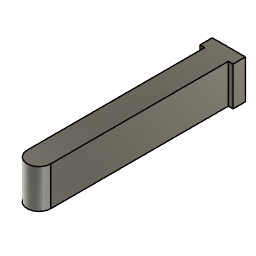
ArcadeSwitchReplacement v3 (Autodesk Fusion 360 design; units mm, degrees)
Autodesk Fusion 360 part; units mm, degrees
sketch "Sketch1" plane through (0, 0, 0) normal (0, 0, 1) x (1, 0, 0)
  line L0 (0, 0) -> (-1.75, 0)
  line L1 (-1.75, 0) -> (-1.75, -1.3)
  line L2 (-1.75, -1.3) -> (-1.25, -1.3)
  line L3 (-1.25, -1.3) -> (-1.25, -21.3)
  line L4 (-1.25, -21.3) -> (1.25, -21.3)
  line L5 (1.25, -21.3) -> (1.25, -1.3)
  line L6 (1.25, -1.3) -> (1.75, -1.3)
  line L7 (1.75, -1.3) -> (1.75, 0)
  line L8 (1.75, 0) -> (0, 0)
  line L9 (1.25, -1.3) -> (-1.25, -1.3) construction
  dimension "d1" = 3.5
  dimension "d2" = 1.3
  dimension "d3" = 20
  dimension "d4" = 2.5
  constraint coincident L0.start L8.end
  constraint horizontal L0
  constraint perpendicular L0 L1
  constraint perpendicular L1 L2
  constraint perpendicular L2 L3
  constraint perpendicular L3 L4
  constraint perpendicular L4 L5
  constraint perpendicular L5 L6
  constraint perpendicular L6 L7
  constraint perpendicular L7 L8
  constraint equal L0 L8
  constraint parallel L2 L9
  constraint equal L2 L6
  measures "d1" distance of L0.end L7.end
  measures "d2" distance of L0.end L1.end
  measures "d3" distance of L2.end L3.end
  measures "d4" distance of L3.end L4.end
extrude "Extrude1" add sketch "Sketch1" along normal blind 4.1
fillet "Fillet1" radius 1.25 2 edges at (1.25, -21.3, 2.05) (-1.25, -21.3, 2.05)
named bodies: "ArcadeSwitchReplacement"
